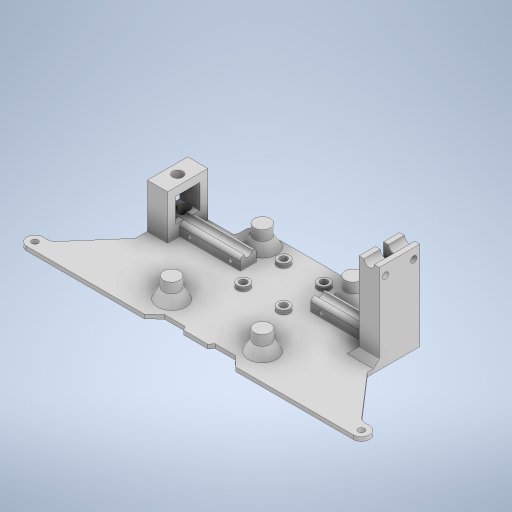
# Autodesk Inventor part: ElectronicsMount - BoltOnStyle
Saved by Autodesk Inventor 2023 (Build 270158000, 158)
## iProperties
Created: 2022-12-11
Part Number: ElectronicsMount - BoltOnStyle
Material: Generic
Document SubType Name: Modeling
Designer: Administrator
Density: 1 g/cm^3
Appearance: Default
Author: Administrator
Autodesk Inventor part; units mm, degrees
note: some values were not read from the file. Chosen so that the rebuilt part matches the saved one: second side of "Extrusion5"; second side of "Extrusion6".
ref_plane "YZ Plane" through (0, 0, 0) normal (1, 0, 0) x (0, 1, 0)
ref_plane "XZ Plane" through (0, 0, 0) normal (0, 1, 0) x (-1, 0, 0)
ref_plane "XY Plane" through (0, 0, 0) normal (0, 0, 1) x (1, 0, 0)
sketch "Sketch1" plane through (0, 0, 0) normal (0, 1, 0) x (-1, 0, 0)
  circle A0 centre (-13, 3.6355) radius 1.25
  circle A1 centre (47, 3.6355) radius 1.25
  circle A2 centre (-63.9, 60.95) radius 1.55
  circle A3 centre (-63.9, 60.95) radius 1.5
  circle A4 centre (97.9, 60.95) radius 1.55
  circle A5 centre (97.9, 60.95) radius 1.5
  arc A6 (47, -0.3645) -> (51, 3.6355) centre (47, 3.6355) ccw
  arc A7 (-17, 3.6355) -> (-13, -0.3645) centre (-13, 3.6355) ccw
  arc A8 (-63.9, 64.95) -> (-63.9, 56.95) centre (-63.9, 60.95) ccw
  arc A9 (97.9, 56.95) -> (97.9, 64.95) centre (97.9, 60.95) ccw
  line L0 (-13, -0.3645) -> (47, -0.3645)
  line L1 (-63.9, 64.95) -> (97.9, 64.95)
  line L2 (-17, 3.6355) -> (-17, 6.1391)
  line L3 (51, 3.6355) -> (51, 6.1391)
  arc A10 (51, 3.6355) -> (47, -0.3645) centre (47, 3.6355) ccw construction
  arc A11 (-13, -0.3645) -> (-17, 3.6355) centre (-13, 3.6355) ccw construction
  line L4 (-63.9, 56.95) -> (-61.722, 56.95)
  line L5 (97.9, 56.95) -> (95.722, 56.95)
  line L6 (92.7041, 55.5753) -> (51.9821, 8.7645)
  line L7 (-58.7041, 55.5753) -> (-17.9821, 8.7645)
  arc A12 (-58.7041, 55.5753) -> (-61.722, 56.95) centre (-61.722, 52.95) ccw
  arc A13 (95.722, 56.95) -> (92.7041, 55.5753) centre (95.722, 52.95) ccw
  arc A14 (51.9821, 8.7645) -> (51, 6.1391) centre (55, 6.1391) ccw
  arc A15 (-17, 6.1391) -> (-17.9821, 8.7645) centre (-21, 6.1391) ccw
  arc A16 (-63.9, 56.95) -> (-63.9, 64.95) centre (-63.9, 60.95) ccw construction
  arc A17 (97.9, 64.95) -> (97.9, 56.95) centre (97.9, 60.95) ccw construction
  point P0 (0, 0)
  point P1 (17, 90.5)
  dimension "d0" = 2.5
  dimension "d1" = 2.5
  dimension "d2" = 3
  dimension "d3" = 3
  dimension "d4" = 8
  dimension "d5" = 8
  dimension "d6" = 8
  dimension "d7" = 8
  dimension "d8" = 60
  dimension "d18" = 4
  constraints: 24 point on circle, 18 centre point, 16 end point, 10 tangent, 5 coincident, 3 equal radius, 2 horizontal, 2 vertical
  measures "d0" diameter of A0
  measures "d1" diameter of A1
  measures "d2" diameter of A3
  measures "d3" diameter of A5
  measures "d4" diameter of A6
  measures "d5" diameter of A7
  measures "d6" diameter of A8
  measures "d7" diameter of A9
  measures "d8" distance of A1.centre A0.centre
  measures "d18" radius of A12
extrude "Extrusion1" add sketch "Sketch1" along normal blind 2 contours L0 A7 L2 A15 L7 A12 L4 A8 L1 A9 L5 A13 L6 A14 L3 A6
sketch "Sketch2" plane through (0, 2, 0) normal (0, 1, 0) x (1, 0, 0)
  circle A0 centre (13, -3.6355) radius 1.25 projected
  circle A1 centre (-47, -3.6355) radius 1.25 projected
  circle A2 centre (-39.5, -6.6355) radius 4
  circle A3 centre (5.5, -6.6355) radius 4
  circle A4 centre (5.5, -51.6355) radius 4
  circle A5 centre (-39.5, -51.6355) radius 4
  line L0 (13, 0.3645) -> (-47, 0.3645) projected
  point P0 (0, 0)
  dimension "d21" = 60
  dimension "d22" = 8
  dimension "d23" = 8
  dimension "d24" = 8
  dimension "d25" = 8
  dimension "d26" = 45
  dimension "d27" = 45
  dimension "d28" = 45
  dimension "d29" = 7
  dimension "d30" = 45
  dimension "d31" = 7.5
  constraints: 4 centre point, 1 horizontal alignment, 1 vertical alignment
  measures "d21" distance of A0.centre A1.centre
  measures "d22" diameter of A2
  measures "d23" diameter of A3
  measures "d24" diameter of A4
  measures "d25" diameter of A5
  measures "d26" distance of A3.centre A2.centre
  measures "d27" distance of A2.centre A5.centre
  measures "d28" distance of A4.centre A5.centre
  measures "d29" distance from line of A3.centre L0
  measures "d30" distance of A4.centre A3.centre
  measures "d31" horizontal distance of A0.centre A3.centre
extrude "Extrusion2" add sketch "Sketch2" along normal blind 10 contours A2 | A3 | A4 | A5
sketch "Sketch3" plane through (0, 2, 0) normal (0, 1, 0) x (1, 0, 0)
  circle A0 centre (13, -3.6355) radius 1.55 construction
  line L0 (13, -3.6355) -> (-2, 2) construction
  line L1 (-2, 2) -> (-2, 4) construction
  line L2 (-2, 2) -> (-2, 4) construction
  line L3 (-2, 4) -> (6, 6.8723) construction
  line L4 (9.8, 6.8723) -> (53.9673, -18.6277) construction
  line L5 (6, 6.8723) -> (9.8, 6.8723) construction
  line L6 (9.8, 6.8723) -> (53.9673, -18.6277) construction
  line L7 (57.4673, -24.6899) -> (57.0036, -33.6779) construction
  line L8 (53.9673, -18.6277) -> (57.4673, -24.6899) construction
  line L9 (57.4673, -24.6899) -> (57.0036, -33.6779) construction
  line L10 (75.376, -65.5) -> (80.5, -65.5) construction
  line L11 (57.0036, -33.6779) -> (75.376, -65.5) construction
  line L12 (75.376, -65.5) -> (6.5, -65.7) construction
  line L13 (6.5, -65.7) -> (6.2893, -65.5) construction
  line L14 (0.6, -60.1) -> (-9.5, -60.1)
  line L15 (-9.5, -60.1) -> (-11, -62.1)
  line L16 (-9.5, -60.1) -> (-11, -62.1)
  line L17 (-23, -62.1) -> (-11, -62.1)
  line L18 (-11, -62.1) -> (-23, -62.1)
  line L19 (-24.5, -60.1) -> (-23, -62.1)
  line L20 (-23, -62.1) -> (-24.5, -60.1)
  line L21 (-34.6, -60.1) -> (-24.5, -60.1)
  line L22 (-24.5, -60.1) -> (-34.6, -60.1)
  line L23 (-40.5, -71.9) -> (-40.5, -65.7) construction
  line L24 (-34.6, -60.1) -> (-39.7098, -64.95)
  line L25 (-114.5, -65.5) -> (-109.376, -65.5) construction
  line L26 (-40.5, -65.7) -> (-109.376, -65.5) construction
  line L27 (-109.376, -65.5) -> (-91.0036, -33.6779) construction
  line L28 (-87.9673, -18.6277) -> (-91.4673, -24.6899) construction
  line L29 (-91.0036, -33.6779) -> (-91.4673, -24.6899) construction
  line L30 (-91.4673, -24.6899) -> (-87.9673, -18.6277) construction
  line L31 (-40, 6.8723) -> (-43.8, 6.8723) construction
  line L32 (-87.9673, -18.6277) -> (-43.8, 6.8723) construction
  line L33 (-43.8, 6.8723) -> (-40, 6.8723) construction
  line L34 (-32, 4) -> (-40, 6.8723) construction
  line L35 (-40, 6.8723) -> (-32, 4) construction
  line L36 (-32, 4) -> (-32, 2) construction
  line L37 (-32, 2) -> (-2, 2) construction
  line L38 (-6.4, -15.5) -> (-2.8831, -15.5)
  line L39 (-2.8831, -15.5) -> (-6.4, -15.5)
  line L40 (-26.1, -17.5) -> (-7.9, -17.5)
  line L41 (-6.4, -15.5) -> (-7.9, -17.5)
  line L42 (-7.9, -17.5) -> (-26.1, -17.5)
  line L43 (-31.1169, -15.5) -> (-27.6, -15.5)
  line L44 (-26.1, -17.5) -> (-27.6, -15.5)
  line L45 (-35.1306, -20.7029) -> (-31.1169, -15.5)
  line L46 (-27.6, -15.5) -> (-31.1169, -15.5)
  line L47 (-31.1169, -15.5) -> (-35.1306, -20.7029)
  line L48 (-35.1306, -20.7029) -> (-27.0449, -36)
  line L49 (-22.7189, -36) -> (-27.0449, -36)
  line L50 (-27.0449, -36) -> (-22.7189, -36)
  line L51 (-20.9689, -37) -> (-22.7189, -36)
  line L52 (-22.7189, -36) -> (-20.9689, -37)
  line L53 (-13.0311, -37) -> (-20.9689, -37)
  line L54 (-20.9689, -37) -> (-13.0311, -37)
  line L55 (-11.2811, -36) -> (-13.0311, -37)
  line L56 (-13.0311, -37) -> (-11.2811, -36)
  line L57 (-6.9551, -36) -> (-11.2811, -36)
  line L58 (-11.2811, -36) -> (-6.9551, -36)
  line L59 (1.1306, -20.7029) -> (-6.9551, -36)
  line L60 (-6.9551, -36) -> (1.1306, -20.7029)
  line L61 (1.1306, -20.7029) -> (-2.8831, -15.5)
  circle A1 centre (13, -3.6355) radius 1.25 projected
  line L62 (-97.9, -64.95) -> (63.9, -64.95) projected
  line L63 (5.7098, -64.95) -> (-39.7098, -64.95)
  line L64 (5.7098, -64.95) -> (0.6, -60.1)
  point P0 (0, 0)
  point P1 (17, 90.5)
  constraints: 128 end point, 15 collinear, 5 perpendicular, 4 parallel, 3 point on line, 1 centre point, 1 coincident
extrude "Extrusion3" cut sketch "Sketch3" against normal up to next contours L64 L62 L24 L21 L19 L17 L15 L14
sketch "Sketch4" plane through (0, 2, 0) normal (0, 1, 0) x (1, 0, 0)
  line L0 (-7, -8.6355) -> (-27, -8.6355) construction
  line L1 (-27, -8.6355) -> (-27, -28.6355) construction
  line L2 (-27, -28.6355) -> (-7, -28.6355) construction
  line L3 (-7, -28.6355) -> (-7, -8.6355) construction
  circle A0 centre (-7, -28.6355) radius 3
  circle A1 centre (-7, -8.6355) radius 3
  circle A2 centre (-27, -8.6355) radius 3
  circle A3 centre (-27, -28.6355) radius 3
  circle A4 centre (13, -3.6355) radius 1.25 projected
  circle A5 centre (-47, -3.6355) radius 1.25 projected
  point P0 (0, 0)
  dimension "d40" = 20
  dimension "d41" = 20
  dimension "d42" = 6
  dimension "d43" = 6
  dimension "d44" = 6
  dimension "d45" = 6
  dimension "d51" = 60
  dimension "d52" = 20
  dimension "d53" = 5
  constraints: 8 end point, 4 centre point, 4 coincident, 2 parallel, 1 horizontal, 1 perpendicular
  measures "d40" distance of L2.end L1.end
  measures "d41" distance of L1.end L0.end
  measures "d42" diameter of A0
  measures "d43" diameter of A1
  measures "d44" diameter of A2
  measures "d45" diameter of A3
  measures "d51" distance of A4.centre A5.centre
  measures "d52" horizontal distance of A5.centre L0.end
  measures "d53" vertical distance of A5.centre L0.end
extrude "Extrusion4" add sketch "Sketch4" along normal blind 2 contours A0 | A1 | A2 | A3
sketch "Sketch5" plane through (0, 2, 0) normal (0, 1, 0) x (1, 0, 0)
  circle A0 centre (-27, -8.6355) radius 3 construction
  line L0 (-27, -8.6355) -> (40.5, -8.6355) construction
  line L1 (40.5, -8.6355) -> (15.5, -8.6355)
  line L2 (15.5, -8.6355) -> (15.5, -38.6355)
  line L3 (15.5, -38.6355) -> (40.5, -38.6355)
  line L4 (40.5, -38.6355) -> (40.5, -8.6355)
  point P0 (0, 0)
  dimension "d48" = 67.5
  dimension "d49" = 25
  dimension "d50" = 30
  constraints: 10 end point, 2 horizontal, 2 parallel, 1 perpendicular
  measures "d48" distance of L0.start L0.end
  measures "d49" distance of L3.end L2.end
  measures "d50" distance of L2.end L1.end
extrude "Extrusion5" add sketch "Sketch5" against normal blind 2
sketch "Sketch6" plane through (0, 2, 0) normal (0, 1, 0) x (1, 0, 0)
  circle A0 centre (-7, -8.6355) radius 3 construction
  line L0 (-7, -8.6355) -> (-74.5, -8.6355) construction
  arc A1 (-51.9821, -8.7645) -> (-51, -6.1391) centre (-55, -6.1391) ccw projected
  line L1 (-51.9821, -8.7645) -> (-92.7041, -55.5753) projected
  line L2 (-74.5, -8.6355) -> (-49.5, -8.6355)
  line L3 (-49.5, -8.6355) -> (-49.5, -38.6355)
  line L4 (-49.5, -38.6355) -> (-74.5, -38.6355)
  line L5 (-74.5, -38.6355) -> (-74.5, -8.6355)
  point P0 (0, 0)
  point P1 (-69.2685, -28.6355)
  point P2 (-51.8746, -8.6355)
  point P3 (-74.5, -34.6493)
  dimension "d58" = 67.5
  dimension "d65" = 25
  dimension "d66" = 30
  constraints: 10 end point, 2 horizontal, 2 parallel, 1 perpendicular
  measures "d58" distance of L0.start L0.end
  measures "d65" distance of L3.end L4.end
  measures "d66" distance of L2.end L3.end
extrude "Extrusion6" add sketch "Sketch6" against normal blind 2
sketch "Sketch7" plane through (0, 2, 0) normal (0, 1, 0) x (1, 0, 0)
  line L0 (40.5, -8.6355) -> (40.5, -34.6493) projected
  line L1 (40.5, -8.6355) -> (30.5, -8.6355)
  line L2 (30.5, -8.6355) -> (30.5, -28.6355)
  line L3 (30.5, -28.6355) -> (40.5, -28.6355)
  line L4 (40.5, -28.6355) -> (40.5, -8.6355)
  point P0 (0, 0)
  dimension "d67" = 10
  dimension "d68" = 20
  constraints: 8 end point, 2 parallel, 1 horizontal, 1 perpendicular
  measures "d67" distance of L3.end L2.end
  measures "d68" distance of L2.end L1.end
extrude "Extrusion7" add sketch "Sketch7" along normal blind 42
sketch "Sketch8" plane through (30.5, 2, 8.6355) normal (-1, 0, 0) x (0, 0, 1)
  line L0 (0, -2) -> (0, 42) construction
  line L1 (0, 42) -> (8, 42) construction
  line L2 (0, 42) -> (20, 42) construction
  line L3 (8, 42) -> (12, 42)
  line L4 (12, 42) -> (12, 2)
  line L5 (12, 2) -> (8, 2)
  line L6 (8, 2) -> (8, 42)
  point P0 (-8.6355, -2)
  dimension "d71" = 8
  dimension "d72" = 4
  dimension "d73" = 40
  constraints: 10 end point, 2 parallel, 1 horizontal, 1 perpendicular, 1 point on line
  measures "d71" distance of L0.end L1.end
  measures "d72" distance of L4.end L5.end
  measures "d73" distance of L3.end L4.end
extrude "Extrusion8" cut sketch "Sketch8" against normal blind 7.5
sketch "Sketch9" plane through (30.5, 2, 28.6355) normal (0, 0, 1) x (1, 0, 0)
  line L0 (0, 0) -> (0, 42) construction
  line L1 (0, 42) -> (5, 42) construction
  line L2 (7.5, 42) -> (0, 42) construction
  circle A0 centre (5, 42) radius 2.5
  point P0 (-30.5, -2)
  dimension "d76" = 5
  dimension "d77" = 5
  constraints: 2 end point, 1 centre point, 1 coincident, 1 point on line
  measures "d76" distance of L0.end L1.end
  measures "d77" diameter of A0
extrude "Extrusion9" cut sketch "Sketch9" against normal up to surface (20 mm away)
sketch "Sketch10" plane through (40.5, 0, 34.6493) normal (1, 0, 0) x (0, 0, -1)
  line L0 (6.0138, 44) -> (26.0138, 44) construction
  line L1 (6.0138, 44) -> (6.0138, 39) construction
  line L2 (6.0138, 2) -> (6.0138, 44) construction
  line L3 (6.0138, 39) -> (9.0138, 39) construction
  line L4 (9.0138, 39) -> (23.0138, 39) construction
  circle A0 centre (9.0138, 39) radius 1.5
  circle A1 centre (23.0138, 39) radius 1.5
  point P0 (34.6493, 0)
  dimension "d80" = 5
  dimension "d81" = 3
  dimension "d82" = 14
  dimension "d83" = 3
  dimension "d84" = 3
  constraints: 6 end point, 2 centre point, 2 coincident, 2 point on line, 1 perpendicular
  measures "d80" distance of L0.start L1.end
  measures "d81" distance of L1.end L3.end
  measures "d82" distance of L3.end L4.end
  measures "d83" diameter of A0
  measures "d84" diameter of A1
extrude "Extrusion10" cut sketch "Sketch10" against normal up to surface (10 mm away)
sketch "Sketch11" plane through (0, 2, 0) normal (0, 1, 0) x (1, 0, 0)
  line L0 (30.5, -16.6355) -> (30.5, -14.6355) construction
  line L1 (30.5, -28.6355) -> (30.5, -8.6355) construction
  line L2 (30.5, -14.6355) -> (0.5, -14.6355)
  line L3 (0.5, -14.6355) -> (0.5, -22.6355)
  line L4 (0.5, -22.6355) -> (30.5, -22.6355)
  line L5 (30.5, -22.6355) -> (30.5, -14.6355)
  line L6 (38, -16.6355) -> (30.5, -16.6355)
  line L7 (30.5, -16.6355) -> (30.5, -20.6355)
  line L8 (30.5, -20.6355) -> (38, -20.6355)
  line L9 (38, -20.6355) -> (38, -16.6355)
  circle A0 centre (-27, -8.6355) radius 3 construction
  line L10 (-27, -8.6355) -> (-34.5, -8.6355) construction
  line L11 (-34.5, -8.6355) -> (-34.5, -14.6355) construction
  line L12 (-34.5, -14.6355) -> (-74.5, -14.6355)
  line L13 (-74.5, -14.6355) -> (-74.5, -22.6355)
  line L14 (-74.5, -22.6355) -> (-34.5, -22.6355)
  line L15 (-34.5, -22.6355) -> (-34.5, -14.6355)
  point P0 (0, 0)
  dimension "d87" = 2
  dimension "d88" = 30
  dimension "d89" = 8
  dimension "d138" = 7.5
  dimension "d139" = 6
  dimension "d140" = 40
  dimension "d141" = 8
  constraints: 30 end point, 6 parallel, 4 horizontal, 3 perpendicular, 1 point on line, 1 vertical
  measures "d87" distance of L0.start L0.end
  measures "d88" distance of L4.end L3.end
  measures "d89" distance of L3.end L2.end
  measures "d138" distance of L10.start L10.end
  measures "d139" distance of L10.end L11.end
  measures "d140" distance of L14.end L13.end
  measures "d141" distance of L13.end L12.end
extrude "Extrusion11" add sketch "Sketch11" along normal blind 6
sketch "Sketch12" plane through (0, 8, 0) normal (0, 1, 0) x (1, 0, 0)
  line L0 (0.5, -14.6355) -> (30.5, -14.6355) projected
  line L1 (0.5, -14.6355) -> (0.5, -16.6355) construction
  line L2 (0.5, -22.6355) -> (0.5, -14.6355) projected
  line L3 (33, -20.6355) -> (30.5, -20.6355) projected
  line L4 (0.5, -20.6355) -> (0.5, -16.6355)
  line L5 (33, -20.6355) -> (38, -20.6355) projected
  line L6 (0.5, -16.6355) -> (38, -16.6355)
  line L7 (38, -16.6355) -> (38, -20.6355)
  line L8 (38, -20.6355) -> (0.5, -20.6355)
  line L9 (0.5, -20.6355) -> (0.5, -16.6355)
  line L10 (-34.5, -22.6355) -> (-34.5, -14.6355) projected
  line L11 (-74.5, -14.6355) -> (-74.5, -22.6355) projected
  line L12 (-34.5, -16.6355) -> (-74.5, -16.6355)
  line L13 (-74.5, -16.6355) -> (-74.5, -20.6355)
  line L14 (-74.5, -20.6355) -> (-34.5, -20.6355)
  line L15 (-34.5, -20.6355) -> (-34.5, -16.6355)
  point P0 (0, 0)
  point P1 (30.5, -20.6355)
  dimension "d92" = 2
  constraints: 20 end point, 4 parallel, 3 point on line, 2 horizontal, 2 perpendicular
  measures "d92" distance of L0.start L1.end
extrude "Extrusion12" cut sketch "Sketch12" against normal blind 2
fillet "Fillet1" radius 2 8 edges at (19.25, 6, 16.6355) (19.25, 6, 20.6355) (15.5, 8, 22.6355) (15.5, 8, 14.6355) (-54.5, 6, 16.6355) (-54.5, 6, 20.6355) (-54.5, 8, 14.6355) (-54.5, 8, 22.6355)
sketch "Sketch13" plane through (0.5, 2, 22.6355) normal (0, 0, 1) x (1, 0, 0)
  line L0 (30, 0) -> (0, 0) construction
  line L1 (0, 0) -> (0, 2) construction
  line L2 (0, 0) -> (0, 4) construction
  line L3 (0, 2) -> (5, 2) construction
  line L4 (5, 2) -> (25, 2) construction
  circle A0 centre (5, 2) radius 1
  circle A1 centre (25, 2) radius 1
  line L5 (-35, 0) -> (-75, 0) construction
  line L6 (-35, 0) -> (-35, 2) construction
  line L7 (-35, 0) -> (-35, 4) construction
  line L8 (-35, 2) -> (-40, 2) construction
  line L9 (-40, 2) -> (-60, 2) construction
  circle A2 centre (-60, 2) radius 1
  circle A3 centre (-40, 2) radius 1
  point P0 (-0.5, -2)
  point P1 (0, 6)
  dimension "d96" = 2
  dimension "d97" = 5
  dimension "d98" = 20
  dimension "d161" = 5
  dimension "d162" = 20
  dimension "d163" = 2
  dimension "d164" = 2
  constraints: 12 end point, 4 centre point, 4 coincident, 2 midpoint, 2 perpendicular, 1 collinear, 1 point on line
  measures "d96" distance of L0.end L1.end
  measures "d97" distance of L1.end L3.end
  measures "d98" distance of L3.end L4.end
  measures "d161" distance of L6.end L8.end
  measures "d162" distance of L8.end L9.end
  measures "d163" diameter of A2
  measures "d164" diameter of A3
extrude "Extrusion13" cut sketch "Sketch13" against normal up to surface (8 mm away)
sketch "Sketch14" plane through (0, 2, 0) normal (0, 1, 0) x (1, 0, 0)
  line L0 (-74.5, -34.6493) -> (-74.5, -8.6355) projected
  line L1 (-74.5, -8.6355) -> (-64.5, -8.6355)
  line L2 (-64.5, -8.6355) -> (-64.5, -28.6355)
  line L3 (-64.5, -28.6355) -> (-74.5, -28.6355)
  line L4 (-74.5, -28.6355) -> (-74.5, -8.6355)
  point P0 (0, 0)
  point P1 (-74.5, -28.6355)
  dimension "d101" = 10
  dimension "d102" = 20
  constraints: 8 end point, 2 parallel, 1 horizontal, 1 perpendicular
  measures "d101" distance of L2.end L3.end
  measures "d102" distance of L1.end L2.end
chamfer "Chamfer1" distance 3 angle 45 2 edges at (30.5, 2, 25.6355) (35.5, 2, 28.6355)
sketch "Sketch15" plane through (-27, 4, 8.6355) normal (0, 1, 0) x (1, 0, 0)
  circle A0 centre (0, 0) radius 1.75
  circle A1 centre (20, -20) radius 3 projected
  circle A2 centre (20, -20) radius 1.75
  circle A3 centre (20, 0) radius 3 projected
  circle A4 centre (20, 0) radius 1.75
  circle A5 centre (0, -20) radius 3 projected
  circle A6 centre (0, -20) radius 1.75
  point P0 (27, 8.6355)
  dimension "d108" = 3.5
  dimension "d109" = 3.5
  dimension "d110" = 3.5
  dimension "d111" = 3.5
  constraints: 4 centre point, 3 coincident
  measures "d108" diameter of A0
  measures "d109" diameter of A2
  measures "d110" diameter of A4
  measures "d111" diameter of A6
extrude "Extrusion15" cut sketch "Sketch15" against normal blind 3 contours A0 | A2 | A4 | A6
sketch "Sketch16" plane through (0, 0, 0) normal (0, -1, 0) x (1, 0, 0)
  line L0 (-34.6, 60.1) -> (-39.7098, 64.95) construction
  line L1 (-34.6, 60.1) -> (-34.6, 54) construction
  line L2 (-34.6, 54) -> (-38.1, 54) construction
  circle A0 centre (-38.1, 54) radius 2.5
  circle A1 centre (4.1, 54) radius 2.5
  line L3 (0.6, 60.1) -> (-9.5, 60.1) construction
  point P0 (0, 0)
  dimension "d114" = 6.1
  dimension "d115" = 3.5
  dimension "d116" = 5
  dimension "d117" = 5
  dimension "d118" = 42.2
  dimension "d119" = 6.1
  constraints: 4 end point, 2 centre point, 1 coincident, 1 perpendicular, 1 vertical
  measures "d114" distance of L0.start L1.end
  measures "d115" distance of L1.end L2.end
  measures "d116" diameter of A0
  measures "d117" diameter of A1
  measures "d118" distance of A1.centre L2.end
  measures "d119" distance from line of A1.centre L3
chamfer "Chamfer2" distance 3 distance2 5 4 edges at (-43.5, 2, 51.6355) (1.5, 2, 51.6355) (-43.5, 2, 6.6355) (1.5, 2, 6.6355)
sketch "Sketch17" plane through (0, 2, 0) normal (0, 1, 0) x (1, 0, 0)
  circle A0 centre (13, -3.6355) radius 1.25 projected
  circle A1 centre (13, -3.6355) radius 2.5
  circle A2 centre (-47, -3.6355) radius 1.25 projected
  circle A3 centre (-47, -3.6355) radius 2.5
  point P0 (0, 0)
  dimension "d125" = 5
  dimension "d126" = 5
  constraints: 2 centre point, 2 coincident
  measures "d125" diameter of A1
  measures "d126" diameter of A3
extrude "Extrusion17" cut sketch "Sketch17" along normal blind 2 contours A0 | A1 | A2 | A3
extrude "Extrusion18" cut sketch "Sketch16" against normal blind 2
extrude "Extrusion20" add sketch "Sketch14" along normal blind 22
sketch "Sketch19" plane through (-64.5, 2, 14.6355) normal (1, 0, 0) x (0, 0, -1)
  line L0 (-10, 18) -> (2, 18)
  line L1 (2, 18) -> (2, 6)
  line L2 (2, 6) -> (-2, 6)
  line L3 (-10, 6) -> (-10, 18)
  line L4 (-14, 0) -> (-14, 22) projected
  line L5 (-14, 22) -> (6, 22) projected
  arc A0 (-6, 6) -> (-2, 6) centre (-4, 6) ccw
  line L6 (-2, 6) -> (-6, 6) construction
  line L7 (-6, 6) -> (-10, 6)
  arc A1 (-2, 6) -> (-6, 6) centre (-4, 6) ccw construction
  point P0 (14.6355, -2)
  dimension "d144" = 12
  dimension "d145" = 12
  dimension "d146" = 4
  dimension "d147" = 4
  constraints: 12 end point, 4 parallel, 4 point on circle, 2 centre point, 1 horizontal, 1 perpendicular
  measures "d144" distance of L1.end L3.start
  measures "d145" distance of L0.end L1.end
  measures "d146" distance between parallel lines of L4 L3
  measures "d147" distance between parallel lines of L5 L0
extrude "Extrusion21" cut sketch "Sketch19" against normal up to surface (10 mm away)
sketch "Sketch20" plane through (0, 0, 0) normal (0, -1, 0) x (1, 0, 0)
  line L0 (-74.5, 34.6493) -> (-74.5, 8.6355) construction
  line L1 (-74.5, 8.6355) -> (-64.5, 8.6355) construction
  line L2 (-64.5, 8.6355) -> (-64.5, 28.6355) construction
  line L3 (-64.5, 28.6355) -> (-74.5, 28.6355) construction
  line L4 (-74.5, 28.6355) -> (-74.5, 8.6355) construction
  line L5 (-74.5, 12.6355) -> (-64.5, 12.6355) construction
  line L6 (-64.5, 12.6355) -> (-64.5, 24.6355) construction
  line L7 (-64.5, 24.6355) -> (-74.5, 24.6355) construction
  line L8 (-74.5, 24.6355) -> (-74.5, 12.6355) construction
  line L9 (-69.5, 12.6355) -> (-69.5, 24.6355) construction
  circle A0 centre (-69.5, 15.1355) radius 2.5
  circle A1 centre (-69.5, 22.1355) radius 2.5
  point P0 (0, 0)
  dimension "d150" = 10
  dimension "d151" = 10
  dimension "d152" = 12
  dimension "d153" = 4
  dimension "d154" = 0
  dimension "d155" = 5
  dimension "d156" = 5
  dimension "d157" = 2.5
  dimension "d158" = 2.5
  constraints: 18 end point, 4 parallel, 2 centre point, 2 horizontal, 2 midpoint, 2 perpendicular, 2 point on line
  measures "d150" distance of L3.end L2.end
  measures "d151" distance of L5.start L5.end
  measures "d152" distance of L7.end L5.start
  measures "d153" distance between parallel lines of L1 L5
  measures "d154" distance between parallel lines of L0 L8
  measures "d155" diameter of A0
  measures "d156" diameter of A1
  measures "d157" distance from line of L5 A0.centre
  measures "d158" distance from line of L7 A1.centre
extrude "Extrusion22" cut sketch "Sketch20" against normal up to surface (8 mm away)
sketch "Sketch21" plane through (0, 24, 0) normal (0, 1, 0) x (1, 0, 0)
  line L0 (-74.5, -8.6355) -> (-51.8746, -8.6355) construction
  line L1 (-74.5, -28.6355) -> (-64.5, -28.6355) construction
  line L2 (-74.5, -8.6355) -> (-64.5, -28.6355) construction
  circle A0 centre (-69.5, -18.6355) radius 2.5
  point P0 (0, 0)
  dimension "d165" = 5
  constraints: 2 end point, 1 centre point, 1 midpoint
  measures "d165" diameter of A0
extrude "Extrusion23" cut sketch "Sketch21" against normal up to surface (4 mm away)
equation "\"d31\" = -0.5 * d26 + 0.5 * d21"
equation "\"d52\" = -0.5 * d40 + 0.5 * d51"
body "Solid1"
